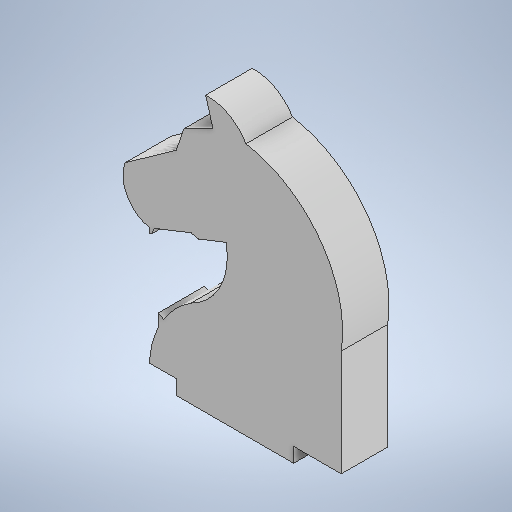
# Autodesk Inventor part: KIGTH TOP abrebotella medium 1.1
Saved by Autodesk Inventor 2025.1 (Build 291241000, 241)
## iProperties
Created: 2024-10-24
Part Number: KIGTH TOP abrebotella medium 1.1
Material: Genérico
Document SubType Name: Modeling
Designer: Octavio
Density: 1 g/cm^3
Appearance: Valor por defecto
Author: Octavio
Autodesk Inventor part; units mm, degrees
ref_plane "YZ Plane" through (0, 0, 0) normal (1, 0, 0) x (0, 1, 0)
ref_plane "XZ Plane" through (0, 0, 0) normal (0, 1, 0) x (-1, 0, 0)
ref_plane "XY Plane" through (0, 0, 0) normal (0, 0, 1) x (1, 0, 0)
sketch "Boceto1" plane through (0, 0, 0) normal (0, 0, 1) x (1, 0, 0)
  line L0 (-55.5895, 69.239) -> (57.1029, 69.239) construction
  line L1 (57.1029, 69.239) -> (57.1029, -41.5752) construction
  line L2 (57.1029, -41.5752) -> (-55.5895, -41.5752) construction
  line L3 (-55.5895, -41.5752) -> (-55.5895, 69.239) construction
  line L4 (-12.6216, 0) -> (12.6216, 0)
  line L5 (12.6216, 0) -> (12.6216, 3.1554)
  line L6 (12.6216, 3.1554) -> (22.8766, 3.1554)
  line L7 (22.8766, 3.1554) -> (22.8766, 26.032)
  arc A0 (22.8766, 26.032) -> (2.3665, 54.4304) centre (-1.924, 29.7261) ccw
  arc A1 (2.3665, 54.4304) -> (-6.3108, 59.1635) centre (-5.9164, 49.5659) ccw
  line L8 (-6.3108, 59.1635) -> (-4.7331, 53.6416)
  line L9 (-4.7331, 53.6416) -> (-11.0439, 50.4862)
  line L10 (-11.0439, 50.4862) -> (-12.6216, 45.7531)
  line L11 (-12.6216, 45.7531) -> (-23.6654, 37.8647)
  arc A2 (-23.6654, 37.8647) -> (-18.4064, 28.3985) centre (-16.9879, 35.3805) ccw
  line L12 (-18.4064, 28.3985) -> (-9.4662, 31.9205)
  line L13 (-9.4662, 31.9205) -> (-7.8885, 31.5539)
  line L14 (-7.8885, 31.5539) -> (-1.924, 33.9035)
  arc A3 (-9.4662, 18.8123) -> (-1.924, 33.9035) centre (-15.5194, 31.2678) ccw
  arc A4 (-9.4662, 18.8123) -> (-18.4064, 3.1554) centre (1.3548, 2.2525) ccw
  line L15 (-18.4064, 3.1554) -> (-12.6216, 3.1554)
  line L16 (-12.6216, 3.1554) -> (-12.6216, 0)
  line L17 (-18.4064, 28.3985) -> (-18.4064, 27.4104)
  line L18 (-18.4064, 27.4104) -> (-18.0172, 27.4104)
  line L19 (-18.0172, 27.4104) -> (-17.3546, 28.8128)
  line L20 (-16.5658, 10.6295) -> (-16.5658, 13.4104)
  line L21 (-16.5658, 13.4104) -> (-15.356, 12.8389)
  point P0 (0, 0)
  point P1 (-18.2118, 27.4104)
  dimension "d8" = 14
  constraints: 36 end point, 12 point on circle, 7 perpendicular, 5 centre point, 2 horizontal, 1 midpoint, 1 parallel, 1 point on line, 1 vertical, 2 other
  measures "d8" vertical distance of L20.end point (-18.212, 27.41)
extrude "Extrusión1" add sketch "Boceto1" along normal mid plane 10
